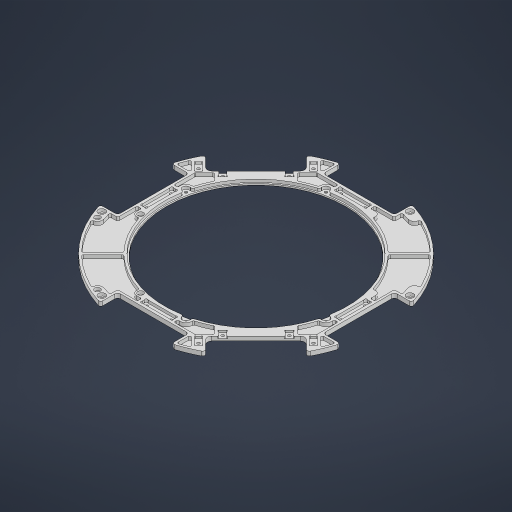
# Autodesk Inventor part: BasePlate
Saved by Autodesk Inventor 2024.2 (Build 282272000, 272)
## iProperties
Created: 2023-12-21
Part Number: BasePlate
Material: 一般
Document SubType Name: Modeling
Designer: Hanaoka
Density: 1 g/cm^3
Appearance: 既定
Author: Hanaoka
Autodesk Inventor part; units mm, degrees
ref_plane "YZ Plane" through (0, 0, 0) normal (1, 0, 0) x (0, 1, 0)
ref_plane "XZ Plane" through (0, 0, 0) normal (0, 1, 0) x (-1, 0, 0)
ref_plane "XY Plane" through (0, 0, 0) normal (0, 0, 1) x (1, 0, 0)
derived "MotorMount_main.ipt"
sketch "モーター固定" plane through (-11, -15, 0) normal (0, -1, 0) x (1, 0, 0)
  circle A0 centre (19.5, 2) radius 0.8
  circle A1 centre (2.5, 2) radius 0.8
  line L0 (22, 0) -> (0, 0)
  line L1 (0, 0) -> (0, 4)
  line L2 (22, 4) -> (0, 4)
  line L3 (22, 0) -> (22, 4)
  circle A2 centre (11, -66) radius 90 construction
  line L4 (2.5, 2) -> (19.5, 2) construction
  line L5 (11, 2) -> (11, -66) construction
  circle A3 centre (11, -66) radius 88
  line L6 (-14, 18.3742) -> (-14, 8)
  line L7 (-12, 6) -> (34, 6)
  line L8 (36, 8) -> (36, 18.3742)
  arc A4 (-14, 8) -> (-12, 6) centre (-12, 8) ccw
  arc A5 (34, 6) -> (36, 8) centre (34, 8) ccw
  line L9 (0, 0) -> (22, 0)
  line L10 (22, 0) -> (22, 4)
  line L11 (22, 4) -> (0, 4)
  line L12 (0, 4) -> (0, 0)
  circle A6 centre (19.5, 2) radius 1
  circle A7 centre (2.5, 2) radius 1
  circle A8 centre (-57, -74.5) radius 1
  line L13 (-59, -77) -> (-55, -77)
  line L14 (-57, -74.5) -> (-57, -57.5) construction
  line L15 (-59, -55) -> (-59, -77)
  line L16 (-55, -55) -> (-59, -55)
  line L17 (-55, -77) -> (-55, -55)
  line L18 (-61, -89) -> (-61, -43)
  circle A9 centre (-57, -57.5) radius 1
  arc A10 (-63, -91) -> (-61, -89) centre (-63, -89) ccw
  line L19 (-63, -41) -> (-73.3742, -41)
  arc A11 (-61, -43) -> (-63, -41) centre (-63, -43) ccw
  line L20 (-73.3742, -91) -> (-63, -91)
  circle A12 centre (19.5, -134) radius 1
  line L21 (22, -136) -> (22, -132)
  line L22 (19.5, -134) -> (2.5, -134) construction
  line L23 (0, -136) -> (22, -136)
  line L24 (0, -132) -> (0, -136)
  line L25 (22, -132) -> (0, -132)
  line L26 (34, -138) -> (-12, -138)
  circle A13 centre (2.5, -134) radius 1
  arc A14 (36, -140) -> (34, -138) centre (34, -140) ccw
  line L27 (-14, -140) -> (-14, -150.3742)
  arc A15 (-12, -138) -> (-14, -140) centre (-12, -140) ccw
  line L28 (36, -150.3742) -> (36, -140)
  circle A16 centre (79, -57.5) radius 1
  line L29 (81, -55) -> (77, -55)
  line L30 (79, -57.5) -> (79, -74.5) construction
  line L31 (81, -77) -> (81, -55)
  line L32 (77, -77) -> (81, -77)
  line L33 (77, -55) -> (77, -77)
  line L34 (83, -43) -> (83, -89)
  circle A17 centre (79, -74.5) radius 1
  arc A18 (85, -41) -> (83, -43) centre (85, -43) ccw
  line L35 (85, -91) -> (95.3742, -91)
  arc A19 (83, -89) -> (85, -91) centre (85, -89) ccw
  line L36 (95.3742, -41) -> (85, -41)
  arc A20 (78.4142, -55) -> (77, -56.4142) centre (77.7071, -55.7071) ccw
  line L37 (77.7071, -55.7071) -> (77.7071, -55) construction
  line L38 (77.7071, -55.7071) -> (77, -55.7071) construction
  line L39 (77.7071, -55.7071) -> (77, -55) construction
  line L40 (80.2929, -55) -> (80.2929, -55.7071) construction
  line L41 (80.2929, -55.7071) -> (81, -55.7071) construction
  line L42 (77.7071, -77) -> (77.7071, -76.2929) construction
  line L43 (77.7071, -76.2929) -> (77, -76.2929) construction
  line L44 (81, -76.2929) -> (80.2929, -76.2929) construction
  line L45 (80.2929, -76.2929) -> (80.2929, -77) construction
  line L46 (81, -77) -> (80.2929, -76.2929) construction
  line L47 (77.7071, -76.2929) -> (77, -77) construction
  line L48 (81, -55) -> (80.2929, -55.7071) construction
  arc A21 (81, -56.4142) -> (79.5858, -55) centre (80.2929, -55.7071) ccw
  arc A22 (79.5858, -77) -> (81, -75.5858) centre (80.2929, -76.2929) ccw
  arc A23 (77, -75.5858) -> (78.4142, -77) centre (77.7071, -76.2929) ccw
  arc A24 (20.5858, 0) -> (22, 1.4142) centre (21.2929, 0.7071) ccw
  arc A25 (22, 2.5858) -> (20.5858, 4) centre (21.2929, 3.2929) ccw
  arc A26 (0, 1.4142) -> (1.4142, 0) centre (0.7071, 0.7071) ccw
  arc A27 (1.4142, 4) -> (0, 2.5858) centre (0.7071, 3.2929) ccw
  arc A28 (-55, -56.4142) -> (-56.4142, -55) centre (-55.7071, -55.7071) ccw
  arc A29 (-57.5858, -55) -> (-59, -56.4142) centre (-58.2929, -55.7071) ccw
  arc A30 (-56.4142, -77) -> (-55, -75.5858) centre (-55.7071, -76.2929) ccw
  arc A31 (-59, -75.5858) -> (-57.5858, -77) centre (-58.2929, -76.2929) ccw
  arc A32 (1.4142, -132) -> (0, -133.4142) centre (0.7071, -132.7071) ccw
  arc A33 (0, -134.5858) -> (1.4142, -136) centre (0.7071, -135.2929) ccw
  arc A34 (22, -133.4142) -> (20.5858, -132) centre (21.2929, -132.7071) ccw
  arc A35 (20.5858, -136) -> (22, -134.5858) centre (21.2929, -135.2929) ccw
  point P0 (11, 0)
  point P1 (-14, 6)
  point P2 (36, 6)
  point P3 (-57, -66)
  point P4 (-61, -91)
  point P5 (-61, -41)
  point P6 (11, -134)
  point P7 (36, -138)
  point P8 (-14, -138)
  point P9 (79, -66)
  point P10 (83, -41)
  point P11 (83, -91)
  point P12 (22, -134.5858)
  point P13 (20.5858, -136)
  point P14 (1.4142, -136)
  point P15 (0, -134.5858)
  point P16 (0, -133.4142)
  point P17 (1.4142, -132)
  point P18 (20.5858, -132)
  point P19 (-59, -75.5858)
  point P20 (-59, -56.4142)
  point P21 (-57.5858, -55)
  point P22 (-55, -75.5858)
  point P23 (0, 2.5858)
  point P24 (1.4142, 4)
  point P25 (20.5858, 4)
  point P26 (22, 2.5858)
  point P27 (22, 1.4142)
  point P28 (20.5858, 0)
  point P29 (1.4142, 0)
  point P30 (0, 1.4142)
  dimension "d4" = 180
  dimension "d5" = 68
  dimension "d6" = 176
  dimension "d11" = 2
  dimension "d12" = 50
  dimension "d13" = 2
  dimension "d14" = 2
  dimension "d17" = 360
  dimension "d31" = 1
  dimension "d32" = 1
  dimension "d35" = 360
  measures "d4" diameter of A2
  measures "d5" distance of L5.start L5.end
  measures "d6" diameter of A3
  measures "d11" distance between parallel lines of L7 L2
  measures "d12" distance of point (-14, 6) point (36, 6)
  measures "d13" radius of A4
  measures "d14" diameter of A7
  measures "d31" radius of A20
  measures "d32" distance of L37.start L29.end
extrude "押し出し2" add sketch "モーター固定" along normal blind 1 contours A24 L0 | L0 L1 L2 L3 | L3 A24 | A26 L0 | L3 A25 | A26 L1 | L2 A25 | A27 L1 | L2 A27 | L36 A18 L34 A19 L35 A3 L28 A14 L26 A15 L27 L20 A10 L18 A11 L19 L6 A4 L7 A5 L8 | A6 | A7 | L15 L16 L17 L13 | A31 L15 | L13 A31 | L13 A30 | A29 L15 | L17 A30 | A29 L16 | L17 A28 | A28 L16 | L23 L24 L25 L21 | A35 L23 | L21 A35 | L21 A34 | A33 L23 | L25 A34 | A33 L24 | L25 A32 | A32 L24 | L31 L32 L33 L29 | A21 L31 | L29 A21 | L29 A20 | A22 L31 | L33 A20 | A22 L32 | L33 A23 | A23 L32
extrude "押し出し3" add sketch "モーター固定" against normal blind 2 contours L36 A18 L34 A19 L35 A3 L28 A14 L26 A15 L27 L20 A10 L18 A11 L19 L6 A4 L7 A5 L8
fillet "フィレット1" radius 1.5 8 edges at (-84.3742, -14.5, -41) (-25, -14.5, 18.3742) (25, -14.5, 18.3742) (84.3742, -14.5, -41) (84.3742, -14.5, -91) (25, -14.5, -150.3742) (-25, -14.5, -150.3742) (-84.3742, -14.5, -91)
sketch "溝切り" plane through (-23, -13, 6) normal (0, 1, 0) x (1, 0, 0)
  circle A0 centre (102.5487, 100.5) radius 2.5
  line L0 (97, 97) -> (105.3408, 97) projected
  arc A1 (106.7686, 98.9595) -> (49.9595, 155.7686) centre (23, 72) ccw projected
  circle A2 centre (102.5487, 100.5) radius 3.5 construction
  line L1 (85.2254, 134.2254) -> (-39.2254, 9.7746) construction
  arc A3 (-60.7686, 45.0405) -> (-3.9595, -11.7686) centre (23, 72) ccw projected
  circle A4 centre (51.5, 151.5487) radius 2.5
  circle A5 centre (51.5, 151.5487) radius 3.5 construction
  line L2 (-39.2254, 134.2254) -> (85.2254, 9.7746) construction
  arc A6 (49.9595, -11.7686) -> (106.7686, 45.0405) centre (23, 72) ccw projected
  arc A7 (-3.9595, 155.7686) -> (-60.7686, 98.9595) centre (23, 72) ccw projected
  circle A8 centre (-5.5, -7.5487) radius 2.5
  circle A9 centre (-5.5, -7.5487) radius 3.5 construction
  circle A10 centre (-56.5487, 43.5) radius 3.5 construction
  circle A11 centre (-56.5487, 43.5) radius 2.5
  circle A12 centre (102.5487, 100.5) radius 1.3
  circle A13 centre (51.5, 151.5487) radius 1.3
  circle A14 centre (-56.5487, 43.5) radius 1.3
  circle A15 centre (-5.5, -7.5487) radius 1.3
  circle A16 centre (23, 72) radius 63
  line L3 (-54.3392, 113.9839) -> (-46.9146, 106.5593)
  line L4 (-42.672, 106.5593) -> (-11.5593, 137.672)
  line L5 (-11.5593, 141.9146) -> (-18.9839, 149.3392)
  arc A17 (-46.9146, 106.5593) -> (-42.672, 106.5593) centre (-44.7933, 108.6806) ccw
  arc A18 (-11.5593, 137.672) -> (-11.5593, 141.9146) centre (-13.6806, 139.7933) ccw
  circle A19 centre (-41.9648, 136.9648) radius 21 construction
  line L6 (64.9839, -5.3392) -> (57.5593, 2.0854)
  line L7 (57.5593, 6.328) -> (88.672, 37.4407)
  line L8 (92.9146, 37.4407) -> (100.3392, 30.0161)
  arc A20 (57.5593, 6.328) -> (57.5593, 2.0854) centre (59.6806, 4.2067) ccw
  arc A21 (92.9146, 37.4407) -> (88.672, 37.4407) centre (90.7933, 35.3194) ccw
  circle A22 centre (8.2657, 135.8212) radius 2.5 construction
  circle A23 centre (8.2657, 135.8212) radius 1
  line L9 (8.2657, 135.8212) -> (23, 72) construction
  arc A24 (10.7016, 136.3836) -> (5.8298, 135.2589) centre (8.2657, 135.8212) ccw
  line L10 (5.8298, 135.2589) -> (6.4033, 132.7746)
  line L11 (10.7016, 136.3836) -> (11.2752, 133.8993)
  circle A25 centre (-40.8212, 86.7343) radius 2.5 construction
  circle A26 centre (-40.8212, 86.7343) radius 1
  arc A27 (-40.2589, 89.1702) -> (-41.3836, 84.2984) centre (-40.8212, 86.7343) ccw
  line L12 (-40.2589, 89.1702) -> (-37.7746, 88.5967)
  line L13 (-41.3836, 84.2984) -> (-38.8993, 83.7248)
  circle A28 centre (86.8212, 57.2657) radius 2.5 construction
  circle A29 centre (86.8212, 57.2657) radius 1
  arc A30 (86.2589, 54.8298) -> (87.3836, 59.7016) centre (86.8212, 57.2657) ccw
  line L14 (86.2589, 54.8298) -> (83.7746, 55.4033)
  line L15 (87.3836, 59.7016) -> (84.8993, 60.2752)
  line L16 (35.2984, 7.6164) -> (34.7248, 10.1007)
  line L17 (40.1702, 8.7411) -> (39.5967, 11.2254)
  circle A31 centre (37.7343, 8.1788) radius 2.5 construction
  circle A32 centre (37.7343, 8.1788) radius 1
  arc A33 (35.2984, 7.6164) -> (40.1702, 8.7411) centre (37.7343, 8.1788) ccw
  circle A34 centre (23, 72) radius 64
  point P0 (23, 6)
  point P1 (-44.7933, 104.4379)
  point P2 (-9.4379, 139.7933)
  point P3 (83.7746, 55.4033)
  point P4 (-37.7746, 88.5967)
  point P5 (-39.8745, 83.95)
  point P6 (34.95, 9.1255)
  point P7 (39.8218, 10.2503)
  point P8 (84.7497, 55.1782)
  point P9 (85.8745, 60.05)
  point P10 (11.05, 134.8745)
  point P11 (6.1782, 133.7497)
  point P12 (-38.7497, 88.8218)
  dimension "d20" = 5
  dimension "d22" = 7
  dimension "d23" = 2.6
  dimension "d28" = 126
  dimension "d37" = 50
  dimension "d38" = 3
  dimension "d39" = 42
  dimension "d40" = 13.5
  dimension "d45" = 2
  dimension "d46" = 5
  dimension "d47" = 32
  dimension "d48" = 1
  constraints: 35 symmetric about line, 34 end point, 31 centre point, 24 point on circle, 18 coincident, 11 tangent, 6 parallel, 5 equal radius, 5 point on line, 1 midpoint, 17 other
  measures "d20" diameter of A0
  measures "d22" diameter of A2
  measures "d23" diameter of A12
  measures "d28" diameter of A16
  measures "d37" distance of point (-44.793, 104.438) point (-9.438, 139.793)
  measures "d38" radius of A17
  measures "d39" diameter of A19
  measures "d40" distance from line of L5.end L4
  measures "d45" diameter of A23
  measures "d46" diameter of A22
  measures "d47" angle of L2 L9
  measures "d48" radial gap between concentric circles of A16 A34
extrude "押し出し4" cut sketch "溝切り" against normal up to surface (3 mm away) contours A12 | A13 | A14 | A15
extrude "押し出し5" cut sketch "溝切り" against normal blind 2 contours A0 | A4 | A8 | A11 | A15 | A16 | A16 L11 A34 L15 | A16 L10 A34 L11 | L15 A34 L14 A16 | A16 L12 A34 L10 | A34 L10 A24 L11 | L14 A34 L17 A16 | L15 A30 L14 A34 | A16 L13 A34 L12 | L17 A34 L16 A16 | A16 L16 A34 L13 | A34 L13 A27 L12 | L17 A33 L16 A34
extrude "押し出し6" cut sketch "溝切り" against normal up to surface (3 mm away) contours L6 A20 L7 A21 L8 A6 | L5 A18 L4 A17 L3 A7 | A16 | A23 | A26 | A29 | A32
fillet "フィレット2" radius 1.5 4 edges at (-77.3392, -14.5, -107.9839) (-41.9839, -14.5, -143.3392) (41.9839, -14.5, 11.3392) (77.3392, -14.5, -24.0161)
fillet "フィレット3" radius 1.5 8 edges at (-61.7497, -14, -82.8218) (-62.8745, -14, -77.95) (-16.8218, -14, -127.7497) (-11.95, -14, -128.8745) (62.8745, -14, -54.05) (61.7497, -14, -49.1782) (11.95, -14, -3.1255) (16.8218, -14, -4.2503)
sketch "シャフト用はめ穴" plane through (-23, -13, -138) normal (0, 1, 0) x (1, 0, 0)
  circle A0 centre (-54.5262, -105.6146) radius 1
  circle A1 centre (-54.5262, -105.6146) radius 2
  circle A2 centre (-41.4205, -88.5) radius 2
  circle A3 centre (-41.4205, -88.5) radius 1
  circle A4 centre (-56.5487, -100.5) radius 2.5 projected
  circle A5 centre (23, -72) radius 63 projected
  arc A6 (-56.5487, -100.5) -> (-54.5262, -105.6146) centre (23, -72) ccw construction
  line L0 (85.2254, -9.7746) -> (-39.2254, -134.2254) construction
  line L1 (-39.2254, -9.7746) -> (85.2254, -134.2254) construction
  circle A7 centre (-10.6146, -149.5262) radius 1
  circle A8 centre (-10.6146, -149.5262) radius 2
  circle A9 centre (-41.4205, -88.5) radius 2.5 construction
  arc A10 (-40.1225, -61.4382) -> (33.5618, -135.1225) centre (23, -72) ccw projected
  line L2 (-44.4142, -83) -> (-45.5858, -83) projected
  circle A11 centre (6.5, -136.4205) radius 2
  circle A12 centre (6.5, -136.4205) radius 1
  circle A13 centre (6.5, -136.4205) radius 2.5 construction
  circle A14 centre (56.6146, 5.5262) radius 1
  circle A15 centre (56.6146, 5.5262) radius 2
  circle A16 centre (39.5, -7.5795) radius 2
  circle A17 centre (39.5, -7.5795) radius 1
  circle A18 centre (100.5262, -38.3854) radius 1
  circle A19 centre (100.5262, -38.3854) radius 2
  circle A20 centre (87.4205, -55.5) radius 2
  circle A21 centre (87.4205, -55.5) radius 1
  point P0 (23, -138)
  dimension "d50" = 2
  dimension "d51" = 4
  dimension "d52" = 1
  dimension "d53" = 5
  dimension "d54" = 3
  constraints: 19 centre point, 13 symmetric about line, 12 coincident, 2 equal radius, 2 point on circle, 1 tangent, 13 other
  measures "d50" diameter of A0
  measures "d51" diameter of A1
  measures "d53" diameter of A9
  measures "d54" distance edge to line of A9 L2
extrude "押し出し7" cut sketch "シャフト用はめ穴" against normal up to surface (2 mm away) contours A0 | A1 | A2 | A3 | A7 | A8 | A11 | A12
extrude "押し出し8" cut sketch "シャフト用はめ穴" against normal up to surface (3 mm away) contours A0 | A3 | A7 | A12
sketch "キッカー用はめあい" plane through (-23, -13, -138) normal (0, 1, 0) x (1, 0, 0)
  circle A0 centre (83.0151, -108.6806) radius 1
  circle A1 centre (59.6806, -132.0151) radius 1
  line L0 (88.672, -106.5593) -> (57.5593, -137.672) projected
  line L1 (73.1156, -122.1156) -> (68.2548, -117.2548) construction
  line L2 (57.5593, -137.672) -> (88.672, -106.5593) projected
  arc A2 (41.1782, -133.3641) -> (84.3641, -90.1782) centre (23, -72) ccw projected
  line L3 (59.6806, -132.0151) -> (83.0151, -108.6806) construction
  line L4 (86.1971, -109.0341) -> (82.6615, -105.4986)
  line L5 (82.6615, -105.4986) -> (79.8331, -108.327)
  line L6 (79.8331, -108.327) -> (83.3687, -111.8626)
  circle A3 centre (83.0151, -108.6806) radius 2 construction
  line L7 (60.0341, -135.1971) -> (56.4986, -131.6615)
  line L8 (56.4986, -131.6615) -> (59.327, -128.8331)
  line L9 (59.327, -128.8331) -> (62.8626, -132.3687)
  arc A4 (83.3687, -106.2057) -> (82.6615, -105.4986) centre (83.0151, -105.8521) ccw
  line L10 (82.6615, -105.4986) -> (83.0151, -105.8521)
  line L11 (79.8331, -108.327) -> (80.1867, -108.6806)
  arc A5 (79.8331, -108.327) -> (80.5402, -109.0341) centre (80.1867, -108.6806) ccw
  arc A6 (56.4986, -131.6615) -> (57.2057, -132.3687) centre (56.8521, -132.0151) ccw
  arc A7 (60.0341, -129.5402) -> (59.327, -128.8331) centre (59.6806, -129.1867) ccw
  line L12 (-21.5477, -116.5477) -> (67.5477, -27.4523) construction
  circle A8 centre (23, -72) radius 63 projected
  circle A9 centre (-13.6806, -11.9849) radius 1
  circle A10 centre (-37.0151, -35.3194) radius 1
  line L13 (-27.1156, -21.8844) -> (-22.2548, -26.7452) construction
  line L14 (-37.0151, -35.3194) -> (-13.6806, -11.9849) construction
  line L15 (-14.0341, -8.8029) -> (-10.4986, -12.3385)
  line L16 (-10.4986, -12.3385) -> (-13.327, -15.1669)
  line L17 (-13.327, -15.1669) -> (-16.8626, -11.6313)
  circle A11 centre (-13.6806, -11.9849) radius 2 construction
  line L18 (-40.1971, -34.9659) -> (-36.6615, -38.5014)
  line L19 (-36.6615, -38.5014) -> (-33.8331, -35.673)
  line L20 (-33.8331, -35.673) -> (-37.3687, -32.1374)
  arc A12 (-10.4986, -12.3385) -> (-11.2057, -11.6313) centre (-10.8521, -11.9849) ccw
  line L21 (-10.4986, -12.3385) -> (-10.8521, -11.9849)
  line L22 (-13.327, -15.1669) -> (-13.6806, -14.8133)
  arc A13 (-14.0341, -14.4598) -> (-13.327, -15.1669) centre (-13.6806, -14.8133) ccw
  arc A14 (-37.3687, -37.7943) -> (-36.6615, -38.5014) centre (-37.0151, -38.1479) ccw
  arc A15 (-33.8331, -35.673) -> (-34.5402, -34.9659) centre (-34.1867, -35.3194) ccw
  line L23 (-40.1971, -34.9659) -> (-37.3687, -32.1374)
  line L24 (-42.672, -37.4407) -> (-11.5593, -6.328) projected
  line L25 (-16.8626, -11.6313) -> (-14.0341, -8.8029)
  line L26 (-54.3392, -37.7943) -> (-51.5108, -34.9659)
  line L27 (-51.5108, -34.9659) -> (-45.8539, -40.6227)
  line L28 (-45.8539, -40.6227) -> (-48.6824, -43.4512)
  line L29 (-48.6824, -43.4512) -> (-54.3392, -37.7943)
  line L30 (-46.9146, -37.4407) -> (-52.9014, -31.454) projected
  line L31 (-11.5593, -6.328) -> (-42.672, -37.4407) projected
  circle A16 centre (-50.0966, -39.2085) radius 1
  line L32 (-51.5108, -40.6227) -> (-48.6824, -37.7943) construction
  line L33 (-47.2681, -42.0369) -> (-52.925, -36.3801) construction
  arc A17 (-53.8392, -37.2943) -> (-53.8392, -38.2943) centre (-53.8392, -37.7943) ccw
  line L34 (-54.3392, -37.7943) -> (-53.8392, -37.7943) construction
  line L35 (-53.8392, -37.7943) -> (-54.0892, -37.5443) construction
  line L36 (-53.8392, -37.7943) -> (-54.0892, -38.0443) construction
  arc A18 (-51.0108, -35.4659) -> (-52.0108, -35.4659) centre (-51.5108, -35.4659) ccw
  arc A19 (-49.1824, -42.9512) -> (-48.1824, -42.9512) centre (-48.6824, -42.9512) ccw
  arc A20 (-46.3539, -41.1227) -> (-46.3539, -40.1227) centre (-46.3539, -40.6227) ccw
  line L37 (-11.2057, 5.3392) -> (-14.0341, 2.5108)
  line L38 (-14.0341, 2.5108) -> (-8.3773, -3.1461)
  line L39 (-8.3773, -3.1461) -> (-5.5488, -0.3176)
  line L40 (-5.5488, -0.3176) -> (-11.2057, 5.3392)
  circle A21 centre (-9.7915, 1.0966) radius 1
  arc A22 (-10.7057, 4.8392) -> (-11.7057, 4.8392) centre (-11.2057, 4.8392) ccw
  arc A23 (-13.5341, 3.0108) -> (-13.5341, 2.0108) centre (-13.5341, 2.5108) ccw
  arc A24 (-6.0488, -0.8176) -> (-6.0488, 0.1824) centre (-6.0488, -0.3176) ccw
  arc A25 (-8.8773, -2.6461) -> (-7.8773, -2.6461) centre (-8.3773, -2.6461) ccw
  line L41 (57.2057, -149.3392) -> (60.0341, -146.5108)
  line L42 (60.0341, -146.5108) -> (54.3773, -140.8539)
  line L43 (54.3773, -140.8539) -> (51.5488, -143.6824)
  line L44 (51.5488, -143.6824) -> (57.2057, -149.3392)
  circle A26 centre (55.7915, -145.0966) radius 1
  arc A27 (56.7057, -148.8392) -> (57.7057, -148.8392) centre (57.2057, -148.8392) ccw
  arc A28 (59.5341, -147.0108) -> (59.5341, -146.0108) centre (59.5341, -146.5108) ccw
  arc A29 (52.0488, -143.1824) -> (52.0488, -144.1824) centre (52.0488, -143.6824) ccw
  arc A30 (54.8773, -141.3539) -> (53.8773, -141.3539) centre (54.3773, -141.3539) ccw
  line L45 (94.6824, -100.5488) -> (100.3392, -106.2057)
  arc A31 (99.8392, -106.7057) -> (99.8392, -105.7057) centre (99.8392, -106.2057) ccw
  line L46 (100.3392, -106.2057) -> (97.5108, -109.0341)
  arc A32 (97.0108, -108.5341) -> (98.0108, -108.5341) centre (97.5108, -108.5341) ccw
  line L47 (97.5108, -109.0341) -> (91.8539, -103.3773)
  circle A33 centre (96.0966, -104.7915) radius 1
  line L48 (91.8539, -103.3773) -> (94.6824, -100.5488)
  arc A34 (95.1824, -101.0488) -> (94.1824, -101.0488) centre (94.6824, -101.0488) ccw
  arc A35 (92.3539, -102.8773) -> (92.3539, -103.8773) centre (92.3539, -103.3773) ccw
  point P0 (23, -138)
  point P1 (56.4986, -131.6615)
  point P2 (57.2057, -132.3687)
  point P3 (-13.327, -15.1669)
  point P4 (-36.6615, -38.5014)
  point P5 (-33.8331, -35.673)
  point P6 (-34.5402, -34.9659)
  point P7 (-37.3687, -37.7943)
  point P8 (-50.0966, -39.2085)
  point P9 (95.1824, -101.0488)
  point P10 (94.1824, -101.0488)
  point P11 (92.3539, -103.8773)
  point P12 (97.0108, -108.5341)
  point P13 (98.0108, -108.5341)
  point P14 (53.8773, -141.3539)
  point P15 (52.0488, -144.1824)
  point P16 (59.5341, -146.0108)
  point P17 (54.8773, -141.3539)
  point P18 (-7.8773, -2.6461)
  point P19 (-6.0488, 0.1824)
  point P20 (-13.5341, 3.0108)
  point P21 (-13.5341, 2.0108)
  point P22 (-8.8773, -2.6461)
  point P23 (-48.1824, -42.9512)
  point P24 (-46.3539, -40.1227)
  point P25 (-51.0108, -35.4659)
  point P26 (-52.0108, -35.4659)
  point P27 (-49.1824, -42.9512)
  dimension "d59" = 2
  dimension "d60" = 33
  dimension "d61" = 2.5
  dimension "d62" = 4
  dimension "d63" = 5
  dimension "d68" = 0.5
  dimension "d69" = 0.5
  dimension "d84" = 8
  dimension "d85" = 4
  dimension "d86" = 1.5
  dimension "d88" = 2
  dimension "d89" = 0.5
  dimension "d90" = 0.5
  constraints: 100 symmetric about line, 88 end point, 51 point on circle, 34 centre point, 33 point on line, 8 coincident, 7 midpoint, 7 parallel, 7 perpendicular, 2 collinear, 2 equal radius, 2 tangent, 1 horizontal, 28 other
  measures "d59" diameter of A0
  measures "d60" distance of L3.start L3.end
  measures "d61" distance between parallel lines of L0 L3
  measures "d62" diameter of A3
  measures "d63" distance of L4.start L4.end
  measures "d68" distance of L4.end L10.end
  measures "d69" radius of A4
  measures "d84" distance of L28.end L29.end
  measures "d85" distance of L26.start L26.end
  measures "d86" distance between parallel lines of L30 L27
  measures "d88" diameter of A16
  measures "d89" distance of L26.start L34.end
  measures "d90" radius of A17
extrude "押し出し9" cut sketch "キッカー用はめあい" against normal blind 1.5 contours A0 | A1 | L0 L6 L5 L4 | L4 A4 | A5 L6 | L0 L7 L8 L9 | L9 A7 | A6 L7 | A9 | A10 | L15 L16 L17 L24 | A12 L15 | L17 A13 | L23 L20 L19 L18 | L18 A14 | A15 L20 | A17 L26 | L26 L27 L28 L29 | L29 A17 | A18 L26 | L29 A19 | A18 L27 | L28 A19 | A20 L27 | L28 A20 | A16 | L40 L39 L38 L37 | A22 L40 | L37 A22 | L37 A23 | A24 L40 | L38 A23 | A24 L39 | L38 A25 | A25 L39 | A21 | L44 L43 L42 L41 | A27 L44 | L41 A27 | L41 A28 | A29 L44 | L42 A28 | A29 L43 | L42 A30 | A30 L43 | A26 | A34 L45 | L45 L46 L47 L48 | L48 A34 | A31 L45 | L48 A35 | A31 L46 | L47 A35 | A32 L46 | L47 A32 | A33
extrude "押し出し10" cut sketch "キッカー用はめあい" against normal up to surface (3 mm away) contours A0 | A1 | A9 | A10 | A16 | A21 | A26 | A33
fillet "フィレット4" radius 0.5 8 edges at (37.0341, -13.75, -2.8029) (39.8626, -13.75, -5.6313) (60.3687, -13.75, -26.1374) (63.1971, -13.75, -28.9659) (-63.1971, -13.75, -103.0341) (-60.3687, -13.75, -105.8626) (-39.8626, -13.75, -126.3687) (-37.0341, -13.75, -129.1971)
sketch "肉抜き" plane through (-23, -13, 6) normal (0, 1, 0) x (1, 0, 0)
  circle A0 centre (102.5487, 100.5) radius 2.5 projected
  circle A1 centre (-5.5, -7.5487) radius 2.5 projected
  circle A2 centre (51.5, 151.5487) radius 2.5 projected
  circle A3 centre (-56.5487, 43.5) radius 2.5 projected
  arc A4 (41.1782, 10.6359) -> (40.1427, 8.8603) centre (41.6043, 9.1977) ccw projected
  line L0 (40.1427, 8.8603) -> (40.1702, 8.7411) projected
  arc A5 (35.2984, 7.6164) -> (40.1702, 8.7411) centre (37.7343, 8.1788) ccw projected
  line L1 (35.2984, 7.6164) -> (35.2709, 7.7355) projected
  arc A6 (35.2709, 7.7355) -> (33.5618, 8.8775) centre (33.8093, 7.3981) ccw projected
  arc A7 (-40.1225, 82.5618) -> (33.5618, 8.8775) centre (23, 72) ccw projected
  arc A8 (-40.1225, 82.5618) -> (-41.2645, 84.2709) centre (-41.6019, 82.8093) ccw projected
  line L2 (-41.2645, 84.2709) -> (-41.3836, 84.2984) projected
  arc A9 (-40.2589, 89.1702) -> (-41.3836, 84.2984) centre (-40.8212, 86.7343) ccw projected
  line L3 (-40.2589, 89.1702) -> (-40.1397, 89.1427) projected
  arc A10 (-40.1397, 89.1427) -> (-38.3641, 90.1782) centre (-39.8023, 90.6043) ccw projected
  arc A11 (4.8218, 133.3641) -> (-38.3641, 90.1782) centre (23, 72) ccw projected
  arc A12 (4.8218, 133.3641) -> (5.8573, 135.1397) centre (4.3957, 134.8023) ccw projected
  line L4 (5.8573, 135.1397) -> (5.8298, 135.2589) projected
  arc A13 (10.7016, 136.3836) -> (5.8298, 135.2589) centre (8.2657, 135.8212) ccw projected
  line L5 (10.7016, 136.3836) -> (10.7291, 136.2645) projected
  arc A14 (10.7291, 136.2645) -> (12.4382, 135.1225) centre (12.1907, 136.6019) ccw projected
  arc A15 (86.1225, 61.4382) -> (12.4382, 135.1225) centre (23, 72) ccw projected
  arc A16 (86.1225, 61.4382) -> (87.2645, 59.7291) centre (87.6019, 61.1907) ccw projected
  line L6 (87.2645, 59.7291) -> (87.3836, 59.7016) projected
  arc A17 (86.2589, 54.8298) -> (87.3836, 59.7016) centre (86.8212, 57.2657) ccw projected
  line L7 (86.2589, 54.8298) -> (86.1397, 54.8573) projected
  arc A18 (86.1397, 54.8573) -> (84.3641, 53.8218) centre (85.8023, 53.3957) ccw projected
  arc A19 (41.1782, 10.6359) -> (84.3641, 53.8218) centre (23, 72) ccw projected
  arc A20 (34, 140.5858) -> (32.5858, 142) centre (33.2929, 141.2929) ccw projected
  line L8 (34, 140.5858) -> (34, 139.4142) projected
  arc A21 (32.5858, 138) -> (34, 139.4142) centre (33.2929, 138.7071) ccw projected
  line L9 (32.5858, 138) -> (13.4142, 138) projected
  arc A22 (12, 139.4142) -> (13.4142, 138) centre (12.7071, 138.7071) ccw projected
  line L10 (12, 139.4142) -> (12, 140.5858) projected
  arc A23 (13.4142, 142) -> (12, 140.5858) centre (12.7071, 141.2929) ccw projected
  line L11 (13.4142, 142) -> (32.5858, 142) projected
  arc A24 (-45.5858, 83) -> (-47, 81.5858) centre (-46.2929, 82.2929) ccw projected
  line L12 (-45.5858, 83) -> (-44.4142, 83) projected
  arc A25 (-43, 81.5858) -> (-44.4142, 83) centre (-43.7071, 82.2929) ccw projected
  line L13 (-43, 81.5858) -> (-43, 62.4142) projected
  arc A26 (-44.4142, 61) -> (-43, 62.4142) centre (-43.7071, 61.7071) ccw projected
  line L14 (-44.4142, 61) -> (-45.5858, 61) projected
  arc A27 (-47, 62.4142) -> (-45.5858, 61) centre (-46.2929, 61.7071) ccw projected
  line L15 (-47, 62.4142) -> (-47, 81.5858) projected
  arc A28 (12, 3.4142) -> (13.4142, 2) centre (12.7071, 2.7071) ccw projected
  line L16 (12, 3.4142) -> (12, 4.5858) projected
  arc A29 (13.4142, 6) -> (12, 4.5858) centre (12.7071, 5.2929) ccw projected
  line L17 (13.4142, 6) -> (32.5858, 6) projected
  arc A30 (34, 4.5858) -> (32.5858, 6) centre (33.2929, 5.2929) ccw projected
  line L18 (34, 4.5858) -> (34, 3.4142) projected
  arc A31 (32.5858, 2) -> (34, 3.4142) centre (33.2929, 2.7071) ccw projected
  line L19 (32.5858, 2) -> (13.4142, 2) projected
  arc A32 (90.4142, 83) -> (89, 81.5858) centre (89.7071, 82.2929) ccw projected
  line L20 (90.4142, 83) -> (91.5858, 83) projected
  arc A33 (93, 81.5858) -> (91.5858, 83) centre (92.2929, 82.2929) ccw projected
  line L21 (93, 81.5858) -> (93, 62.4142) projected
  arc A34 (91.5858, 61) -> (93, 62.4142) centre (92.2929, 61.7071) ccw projected
  line L22 (91.5858, 61) -> (90.4142, 61) projected
  arc A35 (89, 62.4142) -> (90.4142, 61) centre (89.7071, 61.7071) ccw projected
  line L23 (89, 62.4142) -> (89, 81.5858) projected
  circle A36 centre (-41.4205, 55.5) radius 2 projected
  circle A37 centre (6.5, 7.5795) radius 2 projected
  circle A38 centre (-54.5262, 38.3854) radius 2 projected
  circle A39 centre (-10.6146, -5.5262) radius 2 projected
  arc A40 (-13.6806, 135.5506) -> (-13.6806, 134.8435) centre (-13.327, 135.1971) ccw projected
  line L24 (-13.6806, 134.8435) -> (-11.2057, 132.3687) projected
  arc A41 (-10.4986, 131.6615) -> (-11.2057, 132.3687) centre (-10.8521, 132.0151) ccw projected
  line L25 (-10.4986, 131.6615) -> (-13.327, 128.8331) projected
  arc A42 (-14.0341, 129.5402) -> (-13.327, 128.8331) centre (-13.6806, 129.1867) ccw projected
  line L26 (-14.0341, 129.5402) -> (-16.509, 132.0151) projected
  arc A43 (-16.509, 132.0151) -> (-17.2161, 132.0151) centre (-16.8626, 131.6615) ccw projected
  line L27 (-17.2161, 132.0151) -> (-37.0151, 112.2161) projected
  arc A44 (-37.0151, 112.2161) -> (-37.0151, 111.509) centre (-36.6615, 111.8626) ccw projected
  line L28 (-37.0151, 111.509) -> (-34.5402, 109.0341) projected
  arc A45 (-33.8331, 108.327) -> (-34.5402, 109.0341) centre (-34.1867, 108.6806) ccw projected
  line L29 (-33.8331, 108.327) -> (-36.6615, 105.4986) projected
  arc A46 (-37.3687, 106.2057) -> (-36.6615, 105.4986) centre (-37.0151, 105.8521) ccw projected
  line L30 (-37.3687, 106.2057) -> (-39.8435, 108.6806) projected
  arc A47 (-39.8435, 108.6806) -> (-40.5506, 108.6806) centre (-40.1971, 108.327) ccw projected
  line L31 (-40.5506, 108.6806) -> (-42.672, 106.5593) projected
  arc A48 (-46.9146, 106.5593) -> (-42.672, 106.5593) centre (-44.7933, 108.6806) ccw projected
  line L32 (-46.9146, 106.5593) -> (-52.9014, 112.546) projected
  arc A49 (-52.9014, 112.546) -> (-55.2966, 112.1701) centre (-53.962, 111.4854) ccw projected
  arc A50 (-55.2966, 112.1701) -> (-60.7686, 98.9595) centre (23, 72) ccw projected
  arc A51 (-60.7686, 98.9595) -> (-59.3408, 97) centre (-59.3408, 98.5) ccw projected
  line L33 (-59.3408, 97) -> (-51, 97) projected
  arc A52 (-49, 95) -> (-51, 97) centre (-51, 95) ccw projected
  line L34 (-49, 95) -> (-49, 49) projected
  arc A53 (-51, 47) -> (-49, 49) centre (-51, 49) ccw projected
  line L35 (-51, 47) -> (-59.3408, 47) projected
  arc A54 (-59.3408, 47) -> (-60.7686, 45.0405) centre (-59.3408, 45.5) ccw projected
  arc A55 (-60.7686, 45.0405) -> (-3.9595, -11.7686) centre (23, 72) ccw projected
  arc A56 (-3.9595, -11.7686) -> (-2, -10.3408) centre (-3.5, -10.3408) ccw projected
  line L36 (-2, -10.3408) -> (-2, -2) projected
  arc A57 (0, 0) -> (-2, -2) centre (0, -2) ccw projected
  line L37 (0, 0) -> (46, 0) projected
  arc A58 (48, -2) -> (46, 0) centre (46, -2) ccw projected
  line L38 (48, -2) -> (48, -10.3408) projected
  arc A59 (48, -10.3408) -> (49.9595, -11.7686) centre (49.5, -10.3408) ccw projected
  arc A60 (49.9595, -11.7686) -> (63.1701, -6.2966) centre (23, 72) ccw projected
  arc A61 (63.1701, -6.2966) -> (63.546, -3.9014) centre (62.4854, -4.962) ccw projected
  line L39 (63.546, -3.9014) -> (57.5593, 2.0854) projected
  arc A62 (57.5593, 6.328) -> (57.5593, 2.0854) centre (59.6806, 4.2067) ccw projected
  line L40 (57.5593, 6.328) -> (59.6806, 8.4494) projected
  arc A63 (59.6806, 8.4494) -> (59.6806, 9.1565) centre (59.327, 8.8029) ccw projected
  line L41 (59.6806, 9.1565) -> (57.2057, 11.6313) projected
  arc A64 (56.4986, 12.3385) -> (57.2057, 11.6313) centre (56.8521, 11.9849) ccw projected
  line L42 (56.4986, 12.3385) -> (59.327, 15.1669) projected
  arc A65 (60.0341, 14.4598) -> (59.327, 15.1669) centre (59.6806, 14.8133) ccw projected
  line L43 (60.0341, 14.4598) -> (62.509, 11.9849) projected
  arc A66 (62.509, 11.9849) -> (63.2161, 11.9849) centre (62.8626, 12.3385) ccw projected
  line L44 (63.2161, 11.9849) -> (83.0151, 31.7839) projected
  arc A67 (83.0151, 31.7839) -> (83.0151, 32.491) centre (82.6615, 32.1374) ccw projected
  line L45 (83.0151, 32.491) -> (80.5402, 34.9659) projected
  arc A68 (79.8331, 35.673) -> (80.5402, 34.9659) centre (80.1867, 35.3194) ccw projected
  line L46 (79.8331, 35.673) -> (82.6615, 38.5014) projected
  arc A69 (83.3687, 37.7943) -> (82.6615, 38.5014) centre (83.0151, 38.1479) ccw projected
  line L47 (83.3687, 37.7943) -> (85.8435, 35.3194) projected
  arc A70 (85.8435, 35.3194) -> (86.5506, 35.3194) centre (86.1971, 35.673) ccw projected
  line L48 (86.5506, 35.3194) -> (88.672, 37.4407) projected
  arc A71 (92.9146, 37.4407) -> (88.672, 37.4407) centre (90.7933, 35.3194) ccw projected
  line L49 (92.9146, 37.4407) -> (98.9014, 31.454) projected
  arc A72 (98.9014, 31.454) -> (101.2966, 31.8299) centre (99.962, 32.5146) ccw projected
  arc A73 (101.2966, 31.8299) -> (106.7686, 45.0405) centre (23, 72) ccw projected
  arc A74 (106.7686, 45.0405) -> (105.3408, 47) centre (105.3408, 45.5) ccw projected
  line L50 (105.3408, 47) -> (97, 47) projected
  arc A75 (95, 49) -> (97, 47) centre (97, 49) ccw projected
  line L51 (95, 49) -> (95, 95) projected
  arc A76 (97, 97) -> (95, 95) centre (97, 95) ccw projected
  line L52 (97, 97) -> (105.3408, 97) projected
  arc A77 (105.3408, 97) -> (106.7686, 98.9595) centre (105.3408, 98.5) ccw projected
  arc A78 (106.7686, 98.9595) -> (49.9595, 155.7686) centre (23, 72) ccw projected
  arc A79 (49.9595, 155.7686) -> (48, 154.3408) centre (49.5, 154.3408) ccw projected
  line L53 (48, 154.3408) -> (48, 146) projected
  arc A80 (46, 144) -> (48, 146) centre (46, 146) ccw projected
  line L54 (46, 144) -> (0, 144) projected
  arc A81 (-2, 146) -> (0, 144) centre (0, 146) ccw projected
  line L55 (-2, 146) -> (-2, 154.3408) projected
  arc A82 (-2, 154.3408) -> (-3.9595, 155.7686) centre (-3.5, 154.3408) ccw projected
  arc A83 (-3.9595, 155.7686) -> (-17.1701, 150.2966) centre (23, 72) ccw projected
  arc A84 (-17.1701, 150.2966) -> (-17.546, 147.9014) centre (-16.4854, 148.962) ccw projected
  line L56 (-17.546, 147.9014) -> (-11.5593, 141.9146) projected
  arc A85 (-11.5593, 137.672) -> (-11.5593, 141.9146) centre (-13.6806, 139.7933) ccw projected
  line L57 (-11.5593, 137.672) -> (-13.6806, 135.5506) projected
  circle A86 centre (-41.4205, 55.5) radius 1 projected
  arc A87 (-44.4205, 55.5) -> (-40.5891, 52.6175) centre (-41.4205, 55.5) ccw
  circle A88 centre (6.5, 7.5795) radius 1 projected
  line L58 (-44.4205, 55.5) -> (-44.4205, 58.2071)
  line L59 (-45.4205, 59.2071) -> (-46.5, 59.2071)
  line L60 (-47.5, 58.2071) -> (-47.5, 46.5)
  line L61 (-24.7084, 25.7058) -> (-38.1482, 12.266)
  arc A89 (-39.3599, 51.9626) -> (-24.6875, 27.0984) centre (23, 72) ccw
  line L62 (-48.5, 45.5) -> (-51.6313, 45.5)
  arc A90 (-54.4798, 33.5405) -> (-39.5788, 12.2828) centre (23, 72) ccw
  circle A91 centre (-56.5487, 43.5) radius 4 construction
  arc A92 (-53.7934, 34.9629) -> (-51.1679, 39.3712) centre (-54.5262, 38.3854) ccw
  line L63 (-52.5908, 44.2183) -> (-51.1679, 39.3712)
  arc A93 (-60.7686, 45.0405) -> (-3.9595, -11.7686) centre (23, 72) ccw projected
  line L64 (-39.2254, 9.7746) -> (-22.2548, 26.7452) construction
  arc A94 (-46.5, 59.2071) -> (-47.5, 58.2071) centre (-46.5, 58.2071) ccw
  arc A95 (-44.4205, 58.2071) -> (-45.4205, 59.2071) centre (-45.4205, 58.2071) ccw
  arc A96 (-39.3599, 51.9626) -> (-40.5891, 52.6175) centre (-40.3119, 51.6567) ccw
  arc A97 (-48.5, 45.5) -> (-47.5, 46.5) centre (-48.5, 46.5) ccw
  arc A98 (-51.6313, 45.5) -> (-52.5908, 44.2183) centre (-51.6313, 44.5) ccw
  arc A99 (-53.7934, 34.9629) -> (-54.4798, 33.5405) centre (-53.5841, 33.9851) ccw
  arc A100 (-24.7084, 25.7058) -> (-24.6875, 27.0984) centre (-25.4155, 26.4129) ccw
  arc A101 (-39.5788, 12.2828) -> (-38.1482, 12.266) centre (-38.8553, 12.9731) ccw
  arc A102 (3.6175, 8.4109) -> (6.5, 4.5795) centre (6.5, 7.5795) ccw
  line L65 (6.5, 4.5795) -> (9.2071, 4.5795)
  line L66 (10.2071, 3.5795) -> (10.2071, 2.5)
  line L67 (9.2071, 1.5) -> (-2.5, 1.5)
  line L68 (-23.2942, 24.2916) -> (-36.734, 10.8518)
  arc A103 (-21.9016, 24.3125) -> (2.9626, 9.6401) centre (23, 72) ccw
  line L69 (-3.5, 0.5) -> (-3.5, -2.6313)
  arc A104 (-36.7172, 9.4212) -> (-15.4595, -5.4798) centre (23, 72) ccw
  arc A105 (-9.6288, -2.1679) -> (-14.0371, -4.7934) centre (-10.6146, -5.5262) ccw
  line L70 (-4.7817, -3.5908) -> (-9.6288, -2.1679)
  arc A106 (9.2071, 1.5) -> (10.2071, 2.5) centre (9.2071, 2.5) ccw
  arc A107 (10.2071, 3.5795) -> (9.2071, 4.5795) centre (9.2071, 3.5795) ccw
  arc A108 (3.6175, 8.4109) -> (2.9626, 9.6401) centre (2.6567, 8.6881) ccw
  arc A109 (-2.5, 1.5) -> (-3.5, 0.5) centre (-2.5, 0.5) ccw
  arc A110 (-4.7817, -3.5908) -> (-3.5, -2.6313) centre (-4.5, -2.6313) ccw
  arc A111 (-15.4595, -5.4798) -> (-14.0371, -4.7934) centre (-15.0149, -4.5841) ccw
  arc A112 (-21.9016, 24.3125) -> (-23.2942, 24.2916) centre (-22.5871, 23.5845) ccw
  arc A113 (-36.734, 10.8518) -> (-36.7172, 9.4212) centre (-36.0269, 10.1447) ccw
  arc A114 (-57.0327, 104.8179) -> (-58.9036, 99.8216) centre (23, 72) ccw
  line L71 (-57.9568, 98.5) -> (-51.169, 98.5)
  line L72 (-59.3408, 97) -> (-51, 97) projected
  line L73 (-55.4004, 105.1456) -> (-50.4619, 100.2071)
  line L74 (-49.1824, 101.0488) -> (-53.8392, 105.7057) projected
  arc A115 (-55.4004, 105.1456) -> (-57.0327, 104.8179) centre (-56.1075, 104.4385) ccw
  arc A116 (-58.9036, 99.8216) -> (-57.9568, 98.5) centre (-57.9568, 99.5) ccw
  arc A117 (-51.169, 98.5) -> (-50.4619, 100.2071) centre (-51.169, 99.5) ccw
  arc A118 (-35.8022, 100.8539) -> (-39.5525, 91.4278) centre (23, 72) ccw
  line L75 (-35.9929, 102.0015) -> (-39.8435, 105.8521)
  arc A119 (-40.5702, 90.7264) -> (-44.7497, 85.9812) centre (-40.8212, 86.7343) ccw
  line L76 (-45.7318, 84.7929) -> (-46.5, 84.7929)
  line L77 (-47.5, 85.7929) -> (-47.5, 99.1957)
  line L78 (-47.2071, 99.9028) -> (-41.2577, 105.8521)
  line L79 (-46.9146, 106.5593) -> (-52.9014, 112.546) projected
  line L80 (-40.5506, 108.6806) -> (-42.672, 106.5593) projected
  arc A120 (-39.8435, 105.8521) -> (-41.2577, 105.8521) centre (-40.5506, 105.145) ccw
  arc A121 (-35.8022, 100.8539) -> (-35.9929, 102.0015) centre (-36.7, 101.2944) ccw
  arc A122 (-47.2071, 99.9028) -> (-47.5, 99.1957) centre (-46.5, 99.1957) ccw
  arc A123 (-47.5, 85.7929) -> (-46.5, 84.7929) centre (-46.5, 85.7929) ccw
  arc A124 (-45.7318, 84.7929) -> (-44.7497, 85.9812) centre (-45.7318, 85.7929) ccw
  arc A125 (-40.5702, 90.7264) -> (-39.5525, 91.4278) centre (-40.5075, 91.7244) ccw
  line L81 (-27.1156, 122.1156) -> (73.1156, 21.8844) construction
  line L82 (-39.2254, 9.7746) -> (85.2254, 134.2254) construction
  arc A126 (-4.8216, 153.9036) -> (-9.8179, 152.0327) centre (23, 72) ccw
  line L83 (-3.5, 152.9568) -> (-3.5, 146.169)
  line L84 (-10.1456, 150.4004) -> (-5.2071, 145.4619)
  arc A127 (-9.8179, 152.0327) -> (-10.1456, 150.4004) centre (-9.4385, 151.1075) ccw
  arc A128 (-3.5, 152.9568) -> (-4.8216, 153.9036) centre (-4.5, 152.9568) ccw
  arc A129 (-5.2071, 145.4619) -> (-3.5, 146.169) centre (-4.5, 146.169) ccw
  arc A130 (3.5722, 134.5525) -> (-5.8539, 130.8022) centre (23, 72) ccw
  line L85 (-7.0015, 130.9929) -> (-10.8521, 134.8435)
  arc A131 (9.0188, 139.7497) -> (4.2736, 135.5702) centre (8.2657, 135.8212) ccw
  line L86 (10.2071, 140.7318) -> (10.2071, 141.5)
  line L87 (9.2071, 142.5) -> (-4.1957, 142.5)
  line L88 (-4.9028, 142.2071) -> (-10.8521, 136.2577)
  arc A132 (-10.8521, 136.2577) -> (-10.8521, 134.8435) centre (-10.145, 135.5506) ccw
  arc A133 (-7.0015, 130.9929) -> (-5.8539, 130.8022) centre (-6.2944, 131.7) ccw
  arc A134 (-4.1957, 142.5) -> (-4.9028, 142.2071) centre (-4.1957, 141.5) ccw
  arc A135 (10.2071, 141.5) -> (9.2071, 142.5) centre (9.2071, 141.5) ccw
  arc A136 (9.0188, 139.7497) -> (10.2071, 140.7318) centre (9.2071, 140.7318) ccw
  arc A137 (3.5722, 134.5525) -> (4.2736, 135.5702) centre (3.2756, 135.5075) ccw
  arc A138 (50.8216, -9.9036) -> (55.8179, -8.0327) centre (23, 72) ccw
  line L89 (49.5, -8.9568) -> (49.5, -2.169)
  line L90 (56.1456, -6.4004) -> (51.2071, -1.4619)
  arc A139 (55.8179, -8.0327) -> (56.1456, -6.4004) centre (55.4385, -7.1075) ccw
  arc A140 (49.5, -8.9568) -> (50.8216, -9.9036) centre (50.5, -8.9568) ccw
  arc A141 (51.2071, -1.4619) -> (49.5, -2.169) centre (50.5, -2.169) ccw
  arc A142 (42.4278, 9.4475) -> (51.8539, 13.1978) centre (23, 72) ccw
  line L91 (53.0015, 13.0071) -> (56.8521, 9.1565)
  arc A143 (36.9812, 4.2503) -> (41.7264, 8.4298) centre (37.7343, 8.1788) ccw
  line L92 (35.7929, 3.2682) -> (35.7929, 2.5)
  line L93 (36.7929, 1.5) -> (50.1957, 1.5)
  line L94 (50.9028, 1.7929) -> (56.8521, 7.7423)
  arc A144 (56.8521, 7.7423) -> (56.8521, 9.1565) centre (56.145, 8.4494) ccw
  arc A145 (53.0015, 13.0071) -> (51.8539, 13.1978) centre (52.2944, 12.3) ccw
  arc A146 (50.1957, 1.5) -> (50.9028, 1.7929) centre (50.1957, 2.5) ccw
  arc A147 (35.7929, 2.5) -> (36.7929, 1.5) centre (36.7929, 2.5) ccw
  arc A148 (36.9812, 4.2503) -> (35.7929, 3.2682) centre (36.7929, 3.2682) ccw
  arc A149 (42.4278, 9.4475) -> (41.7264, 8.4298) centre (42.7244, 8.4925) ccw
  arc A150 (101.4004, 38.8544) -> (103.0327, 39.1821) centre (102.1075, 39.5615) ccw
  arc A151 (103.0327, 39.1821) -> (104.9036, 44.1784) centre (23, 72) ccw
  arc A152 (104.9036, 44.1784) -> (103.9568, 45.5) centre (103.9568, 44.5) ccw
  line L95 (103.9568, 45.5) -> (97.169, 45.5)
  arc A153 (97.169, 45.5) -> (96.4619, 43.7929) centre (97.169, 44.5) ccw
  line L96 (101.4004, 38.8544) -> (96.4619, 43.7929)
  arc A154 (85.8435, 38.1479) -> (87.2577, 38.1479) centre (86.5506, 38.855) ccw
  line L97 (93.2071, 44.0972) -> (87.2577, 38.1479)
  arc A155 (93.2071, 44.0972) -> (93.5, 44.8043) centre (92.5, 44.8043) ccw
  line L98 (93.5, 58.2071) -> (93.5, 44.8043)
  arc A156 (93.5, 58.2071) -> (92.5, 59.2071) centre (92.5, 58.2071) ccw
  line L99 (91.7318, 59.2071) -> (92.5, 59.2071)
  arc A157 (91.7318, 59.2071) -> (90.7497, 58.0188) centre (91.7318, 58.2071) ccw
  arc A158 (86.5702, 53.2736) -> (85.5525, 52.5722) centre (86.5075, 52.2756) ccw
  arc A159 (86.5702, 53.2736) -> (90.7497, 58.0188) centre (86.8212, 57.2657) ccw
  arc A160 (81.8022, 43.1461) -> (85.5525, 52.5722) centre (23, 72) ccw
  line L100 (81.9929, 41.9985) -> (85.8435, 38.1479)
  arc A161 (81.8022, 43.1461) -> (81.9929, 41.9985) centre (82.7, 42.7056) ccw
  arc A162 (42.3825, 135.5891) -> (39.5, 139.4205) centre (39.5, 136.4205) ccw
  line L101 (39.5, 139.4205) -> (36.7929, 139.4205)
  line L102 (35.7929, 140.4205) -> (35.7929, 141.5)
  line L103 (36.7929, 142.5) -> (48.5, 142.5)
  line L104 (69.2942, 119.7084) -> (82.734, 133.1482)
  arc A163 (67.9016, 119.6875) -> (43.0374, 134.3599) centre (23, 72) ccw
  line L105 (49.5, 143.5) -> (49.5, 146.6313)
  arc A164 (82.7172, 134.5788) -> (61.4595, 149.4798) centre (23, 72) ccw
  arc A165 (55.6288, 146.1679) -> (60.0371, 148.7934) centre (56.6146, 149.5262) ccw
  line L106 (50.7817, 147.5908) -> (55.6288, 146.1679)
  arc A166 (36.7929, 142.5) -> (35.7929, 141.5) centre (36.7929, 141.5) ccw
  arc A167 (35.7929, 140.4205) -> (36.7929, 139.4205) centre (36.7929, 140.4205) ccw
  arc A168 (42.3825, 135.5891) -> (43.0374, 134.3599) centre (43.3433, 135.3119) ccw
  arc A169 (48.5, 142.5) -> (49.5, 143.5) centre (48.5, 143.5) ccw
  arc A170 (50.7817, 147.5908) -> (49.5, 146.6313) centre (50.5, 146.6313) ccw
  arc A171 (61.4595, 149.4798) -> (60.0371, 148.7934) centre (61.0149, 148.5841) ccw
  arc A172 (67.9016, 119.6875) -> (69.2942, 119.7084) centre (68.5871, 120.4155) ccw
  arc A173 (82.734, 133.1482) -> (82.7172, 134.5788) centre (82.0269, 133.8553) ccw
  line L107 (91.4205, 84.7929) -> (92.5, 84.7929)
  arc A174 (92.5, 84.7929) -> (93.5, 85.7929) centre (92.5, 85.7929) ccw
  arc A175 (90.4205, 85.7929) -> (91.4205, 84.7929) centre (91.4205, 85.7929) ccw
  line L108 (90.4205, 88.5) -> (90.4205, 85.7929)
  arc A176 (90.4205, 88.5) -> (86.5891, 91.3825) centre (87.4205, 88.5) ccw
  line L109 (93.5, 85.7929) -> (93.5, 97.5)
  line L110 (94.5, 98.5) -> (97.6313, 98.5)
  arc A177 (94.5, 98.5) -> (93.5, 97.5) centre (94.5, 97.5) ccw
  arc A178 (97.6313, 98.5) -> (98.5908, 99.7817) centre (97.6313, 99.5) ccw
  line L111 (98.5908, 99.7817) -> (97.1679, 104.6288)
  arc A179 (99.7934, 109.0371) -> (97.1679, 104.6288) centre (100.5262, 105.6146) ccw
  arc A180 (99.7934, 109.0371) -> (100.4798, 110.4595) centre (99.5841, 110.0149) ccw
  arc A181 (100.4798, 110.4595) -> (85.5788, 131.7172) centre (23, 72) ccw
  arc A182 (85.5788, 131.7172) -> (84.1482, 131.734) centre (84.8553, 131.0269) ccw
  line L112 (70.7084, 118.2942) -> (84.1482, 131.734)
  arc A183 (70.7084, 118.2942) -> (70.6875, 116.9016) centre (71.4155, 117.5871) ccw
  arc A184 (85.3599, 92.0374) -> (70.6875, 116.9016) centre (23, 72) ccw
  arc A185 (85.3599, 92.0374) -> (86.5891, 91.3825) centre (86.3119, 92.3433) ccw
  point P0 (23, 6)
  point P1 (-24.0172, 26.397)
  point P2 (-38.8678, 11.5465)
  point P3 (-24.0172, 26.397)
  point P4 (-38.8678, 11.5465)
  point P5 (-56.4528, 106.198)
  point P6 (-59.3408, 98.5)
  point P7 (-59.3408, 98.5)
  point P8 (-35.4843, 101.4929)
  point P9 (-44.3185, 84.7929)
  dimension "d71" = 1.5
  dimension "d72" = 3
  dimension "d73" = 1.5
  dimension "d74" = 1.5
  dimension "d75" = 1.5
  dimension "d76" = 8
  dimension "d77" = 1.5
  dimension "d79" = 1.5
  dimension "d80" = 1
  dimension "d81" = 1
  dimension "d91" = 1.5
  dimension "d92" = 1.5
  dimension "d93" = 1.5
  dimension "d94" = 1
  dimension "d95" = 1.5
  dimension "d96" = 1.5
  dimension "d97" = 1.5
  dimension "d98" = 1.5
  dimension "d99" = 1.5
  dimension "d100" = 1.5
  dimension "d101" = 1
  constraints: 211 point on circle, 171 symmetric about line, 102 end point, 97 centre point, 37 tangent, 14 equal radius, 13 point on line, 10 coincident, 5 parallel, 3 horizontal, 3 perpendicular, 2 midpoint, 1 concentric, 1 vertical, 72 other
  measures "d71" radial gap between concentric circles of A7 A89
  measures "d72" radius of A87
  measures "d73" distance edge to line of A27 L59
  measures "d74" distance between parallel lines of L34 L60
  measures "d75" distance between parallel lines of L35 L62
  measures "d76" diameter of A91
  measures "d77" radial gap between concentric circles of A55 A90
  measures "d79" radial gap between concentric circles of A92 A38
  measures "d80" distance between parallel lines of L64 L61
  measures "d81" radius of A94
  measures "d91" radial gap between concentric circles of A50 A114
  measures "d92" distance between parallel lines of L33 L71
  measures "d93" distance between parallel lines of L74 L73
  measures "d94" radius of A115
  measures "d95" radial gap between concentric circles of A118 A11
  measures "d96" radial gap between concentric circles of A119 A9
  measures "d97" distance edge to line of A46 L75
  measures "d98" distance between parallel lines of L34 L77
  measures "d99" distance between parallel lines of L31 L78
  measures "d100" distance edge to line of A24 L76
  measures "d101" radius of A120
extrude "押し出し11" cut sketch "肉抜き" against normal blind 2.5 contours A87 A96 A89 A100 L61 A101 A90 A99 A92 L63 A98 L62 A97 L60 A94 L59 A95 L58 | A102 L65 A107 L66 A106 L67 A109 L69 A110 L70 A105 A111 A104 A113 L68 A112 A103 A108 | A115 L73 A117 L71 A116 A114 | A118 A125 A119 A124 L76 A123 L77 A122 L78 A120 L75 A121 | A128 L83 A129 L84 A127 A126 | A130 A133 L85 A132 L88 A134 L87 A135 L86 A136 A131 A137 | A140 L89 A141 L90 A139 A138 | A142 A145 L91 A144 L94 A146 L93 A147 L92 A148 A143 A149 | L96 A153 L95 A152 A151 A150 | L100 A161 A160 A158 A159 A157 L99 A156 L98 A155 L97 A154 | A162 L101 A167 L102 A166 L103 A169 L105 A170 L106 A165 A171 A164 A173 L104 A172 A163 A168 | A175 L108 A176 A185 A184 A183 L112 A182 A181 A180 A179 L111 A178 L110 A177 L109 A174 L107
